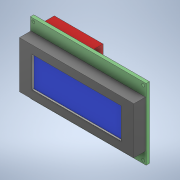
# Autodesk Inventor part: 2020-04-12 LcdAssembly
Saved by Autodesk Inventor 2020 (Build 240168000, 168)
## iProperties
Created: 2019-12-15
Part Number: 2020-04-12 LcdAssembly
Material: Generic
Document SubType Name: Modeling
Designer: torto
Density: 1 g/cm^3
Appearance: Default
Author: torto
Autodesk Inventor part; units mm, degrees
ref_plane "YZ Plane" through (0, 0, 0) normal (1, 0, 0) x (0, 1, 0)
ref_plane "XZ Plane" through (0, 0, 0) normal (0, 1, 0) x (-1, 0, 0)
ref_plane "XY Plane" through (0, 0, 0) normal (0, 0, 1) x (1, 0, 0)
sketch "Sketch1" plane through (0, 0, 0) normal (0, 0, 1) x (1, 0, 0)
  line L0 (0, 0) -> (98.3, 0)
  line L1 (98.3, 0) -> (98.3, 60.2)
  line L2 (98.3, 60.2) -> (0, 60.2)
  line L3 (0, 60.2) -> (0, 0)
  line L4 (0, 60.2) -> (2.5, 60.2) construction
  line L5 (2.5, 60.2) -> (2.5, 57.7) construction
  line L6 (2.5, 57.7) -> (0, 57.7) construction
  line L7 (0, 57.7) -> (0, 60.2) construction
  circle A0 centre (2.5, 57.7) radius 1.25
  line L8 (49.15, 60.2) -> (49.15, 0) construction
  line L9 (0, 30.1) -> (98.3, 30.1) construction
  circle A1 centre (95.8, 57.7) radius 1.25
  circle A2 centre (2.5, 2.5) radius 1.25
  circle A3 centre (95.8, 2.5) radius 1.25
  dimension "d0" = 98.3
  dimension "d1" = 60.2
  dimension "d2" = 2.5
  dimension "d7" = 2.5
  dimension "d8" = 2.5
  constraints: 20 end point, 4 centre point, 4 midpoint, 4 parallel, 3 symmetric about line, 2 horizontal, 2 perpendicular, 1 coincident, 3 other
  measures "d0" distance of L1.end L2.end
  measures "d1" distance of L0.end L1.end
  measures "d2" distance of L4.end L5.end
  measures "d7" distance of L5.end L6.end
  measures "d8" diameter of A0
extrude "LcdPcb" add sketch "Sketch1" along normal blind 2.8
sketch "Sketch2" plane through (0, 0, 2.8) normal (0, 0, 1) x (1, 0, 0)
  line L0 (98.3, 60.2) -> (0, 60.2) construction
  line L1 (49.15, 60.2) -> (49.15, 0) construction
  line L2 (0, 0) -> (98.3, 0) construction
  line L3 (0, 60.2) -> (0, 0) construction
  line L4 (0, 30.1) -> (98.3, 30.1) construction
  line L5 (98.3, 0) -> (98.3, 60.2) construction
  line L6 (0.5, 50) -> (97.8, 50)
  line L7 (97.8, 50) -> (97.8, 10.2)
  line L8 (97.8, 10.2) -> (0.5, 10.2)
  line L9 (0.5, 10.2) -> (0.5, 50)
  line L10 (0.5, 50) -> (97.8, 10.2) construction
  line L11 (97.8, 50) -> (0.5, 10.2) construction
  point P0 (49.15, 30.1)
  dimension "d15" = 39.8
  dimension "d16" = 97.3
  constraints: 16 end point, 7 midpoint, 2 parallel, 1 horizontal, 1 perpendicular
  measures "d15" distance of L6.end L7.end
  measures "d16" distance of L7.end L8.end
extrude "LcdBezel" add sketch "Sketch2" along normal blind 9.9
sketch "Sketch3" plane through (0, 0, 12.7) normal (0, 0, 1) x (1, 0, 0)
  line L0 (0.5, 50) -> (0.5, 10.2) construction
  line L1 (0.5, 50) -> (11.3, 50) construction
  line L2 (11.3, 50) -> (11.3, 43.1) construction
  line L3 (11.3, 43.1) -> (0.5, 43.1) construction
  line L4 (0.5, 43.1) -> (0.5, 50) construction
  line L5 (11.3, 43.1) -> (87, 43.1)
  line L6 (87, 43.1) -> (87, 17.1)
  line L7 (87, 17.1) -> (11.3, 17.1)
  line L8 (11.3, 17.1) -> (11.3, 43.1)
  point P0 (0, 0)
  dimension "LcdBezelHeight" = 6.9
  dimension "LcdBezelLength" = 10.8
  dimension "d28" = 75.7
  dimension "d29" = 26
  constraints: 16 end point, 4 parallel, 2 horizontal, 2 perpendicular
  measures "LcdBezelHeight" distance of L1.end L2.end
  measures "LcdBezelLength" distance of L2.end L3.end
  measures "d28" distance of L6.end L7.end
  measures "d29" distance of L5.end L6.end
extrude "Lcd" cut sketch "Sketch3" against normal blind 1.4
sketch "Sketch4" plane through (0, 0, 0) normal (0, 0, -1) x (-1, 0, 0)
  line L0 (0, 60.2) -> (0, 0) construction
  line L1 (0, 60.2) -> (-7.5, 60.2) construction
  line L2 (-7.5, 60.2) -> (-7.5, 58.2) construction
  line L3 (-7.5, 58.2) -> (0, 58.2) construction
  line L4 (0, 58.2) -> (0, 60.2) construction
  line L5 (-7.5, 58.2) -> (-49, 58.2)
  line L6 (-49, 58.2) -> (-49, 39.2)
  line L7 (-49, 39.2) -> (-7.5, 39.2)
  line L8 (-7.5, 39.2) -> (-7.5, 58.2)
  dimension "LcdRearKeepOutHeightOffset" = 2
  dimension "LcdRearKeepOutLengthOffset" = 7.5
  dimension "LcdRearKeepOutHeight" = 19
  dimension "LcdRearKeepOutLength" = 41.5
  constraints: 16 end point, 4 parallel, 2 horizontal, 2 perpendicular
  measures "LcdRearKeepOutHeightOffset" distance of L1.end L2.end
  measures "LcdRearKeepOutLengthOffset" distance of L2.end L3.end
  measures "LcdRearKeepOutHeight" distance of L5.end L6.end
  measures "LcdRearKeepOutLength" distance of L6.end L7.end
extrude "LcdRearKeepOut" add sketch "Sketch4" along normal blind 10
equation "\"d0\" = LcdBorderLength"
equation "\"d1\" = LcdBorderHeight"
equation "\"d2\" = LcdFrameHoleOffset"
equation "\"d7\" = LcdFrameHoleOffset"
equation "\"d8\" = LcdFrameHoleDiameterUntapped"
equation "\"d12\" = LcdPcbThickness"
equation "\"d15\" = LcdHeight"
equation "\"d16\" = LcdLength"
equation "\"d28\" = LcdLength - 2 * LcdBezelLength"
equation "\"d29\" = LcdHeight - 2 * LcdBezelHeight"
equation "\"d30\" = 0.5 * LcdPcbThickness"
equation "\"LcdBorderLength\" = 98.3"
equation "\"LcdBorderHeight\" = 60.2"
equation "\"LcdFrameHoleOffset\" = 2.5"
equation "\"LcdFrameHoleDiameterUntapped\" = 2.5"
equation "\"LcdPcbThickness\" = 2.8"
equation "\"LcdHeight\" = 39.8"
equation "\"LcdLength\" = 97.3"
body "Solid1"
